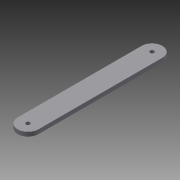
# Autodesk Inventor part: Part4
Saved by Autodesk Inventor 2015 (Build 190159000, 159)
## iProperties
Created: 2014-07-15
Part Number: Part4
Material: Generic
Document SubType Name: Modeling
Designer: shohei
Density: 1 g/cm^3
Appearance: Default
Mass: 167.974 g
Surface Area: 417.902 cm^2
Volume: 167.974 cm^3
Author: shohei
Autodesk Inventor part; units mm, degrees
ref_plane "YZ Plane" through (0, 0, 0) normal (1, 0, 0) x (0, 1, 0)
ref_plane "XZ Plane" through (0, 0, 0) normal (0, 1, 0) x (-1, 0, 0)
ref_plane "XY Plane" through (0, 0, 0) normal (0, 0, 1) x (1, 0, 0)
sketch "Sketch1" plane through (0, 0, 0) normal (0, 0, 1) x (1, 0, 0)
  line L0 (-7.5, 170) -> (7.5, 170)
  line L1 (7.5, 170) -> (7.5, -170)
  line L2 (7.5, -170) -> (-7.5, -170)
  line L3 (-7.5, -170) -> (-7.5, 170)
  line L4 (-10.5, 0) -> (10.5, 0) projected
  line L5 (0, -238) -> (0, 238) projected
  point P0 (0, 0)
  dimension "d4" = 7.5
  dimension "d5" = 7.5
  dimension "d6" = 170
  dimension "d7" = 170
  constraints: 8 end point, 2 parallel, 1 horizontal, 1 perpendicular
  measures "d4" distance between parallel lines of L1 L5
  measures "d5" distance between parallel lines of L3 L5
  measures "d6" distance between parallel lines of L0 L4
  measures "d7" distance between parallel lines of L2 L4
extrude "Extrusion1" add sketch "Sketch1" along normal blind 10
sketch "Sketch2" plane through (0, 0, 10) normal (0, 0, 1) x (1, 0, 0)
  circle A0 centre (0, 150) radius 5
  circle A1 centre (0, -150) radius 5
  line L0 (-10.5, 0) -> (10.5, 0) projected
  line L1 (0, -238) -> (0, 238) projected
  point P0 (0, 0)
  dimension "d8" = 10
  dimension "d9" = 150
  dimension "d10" = 150
  dimension "d11" = 10
  constraints: 2 centre point
  measures "d8" diameter of A0
  measures "d9" distance from line of L0 A0.centre
  measures "d10" distance from line of A1.centre L0
  measures "d11" diameter of A1
extrude "Extrusion2" cut sketch "Sketch2" against normal blind 180
sketch "Sketch3" plane through (0, 0, 10) normal (0, 0, 1) x (1, 0, 0)
  arc A0 (25, 149.8188) -> (-25, 149.8188) centre (0, 149.8188) ccw
  circle A1 centre (0, -150) radius 5 projected
  arc A2 (-25, -150) -> (25, -150) centre (0, -150) ccw
  line L0 (-25, 149.8188) -> (-25, -150)
  line L1 (25, 149.8188) -> (25, -150)
  line L2 (7.5, -170) -> (7.5, 170) projected
  point P0 (0, 0)
  dimension "d12" = 50
  dimension "d13" = 50
  constraints: 4 end point, 4 point on circle, 2 centre point, 1 coincident, 1 parallel, 1 tangent
  measures "d12" diameter of A0
  measures "d13" diameter of A2
extrude "Extrusion3" add sketch "Sketch3" against normal blind 10
mirror "Mirror1" about plane through (0, 0, 0) normal (0, 1, 0) of "Extrusion2"
body "Solid1"
